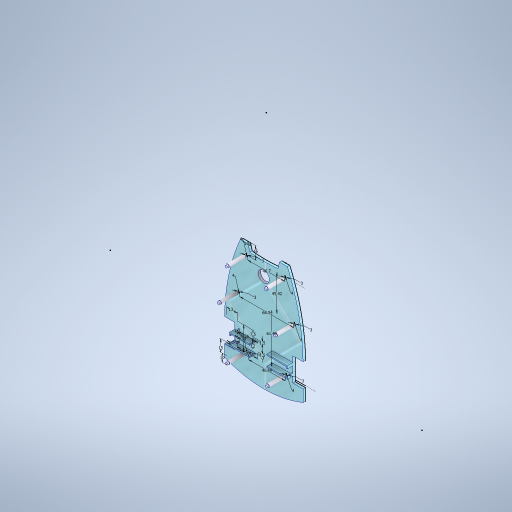
# Autodesk Inventor part: Part1
Saved by Autodesk Inventor 2024 (Build 280153000, 153)
## iProperties
Created: 2024-04-12
Part Number: Part1
Material: Generic
Document SubType Name: Modeling
Designer: Hitesh
Density: 1 g/cm^3
Appearance: Cool White
Author: Hitesh
Autodesk Inventor part; units mm, degrees
ref_plane "YZ Plane" through (0, 0, 0) normal (1, 0, 0) x (0, 1, 0)
ref_plane "XZ Plane" through (0, 0, 0) normal (0, 1, 0) x (-1, 0, 0)
ref_plane "XY Plane" through (0, 0, 0) normal (0, 0, 1) x (1, 0, 0)
sketch "Sketch1" plane through (0, 0, 0) normal (0, 0, 1) x (1, 0, 0)
  arc A0 (0, 10) -> (100, 10) centre (50, 130) ccw
  line L0 (0, 55) -> (13, 55)
  line L1 (13, 55) -> (13, 25)
  line L2 (13, 25) -> (0, 25)
  line L3 (13, 47.5) -> (39, 47.5)
  line L4 (39, 47.5) -> (39, 46)
  line L5 (39, 46) -> (13, 46)
  line L6 (13, 46) -> (13, 47.5)
  line L7 (13, 34) -> (39, 34)
  line L8 (39, 34) -> (39, 32.5)
  line L9 (39, 32.5) -> (13, 32.5)
  line L10 (13, 46) -> (14, 46)
  line L11 (14, 46) -> (14, 44)
  line L12 (14, 44) -> (13, 44)
  line L13 (13, 44) -> (13, 46)
  line L14 (13, 34) -> (14, 34)
  line L15 (14, 34) -> (14, 36)
  line L16 (14, 36) -> (13, 36)
  line L17 (13, 36) -> (13, 34)
  line L18 (30, 150) -> (32, 142)
  arc A1 (32, 142) -> (50, 141) centre (50, 303.5) ccw
  line L19 (100, 55) -> (87, 55)
  line L20 (87, 55) -> (87, 25)
  line L21 (87, 25) -> (100, 25)
  line L22 (87, 47.5) -> (61, 47.5)
  line L23 (61, 47.5) -> (61, 46)
  line L24 (61, 46) -> (87, 46)
  line L25 (87, 46) -> (87, 47.5)
  line L26 (61, 34) -> (61, 32.5)
  line L27 (87, 34) -> (61, 34)
  line L28 (61, 32.5) -> (87, 32.5)
  line L29 (87, 46) -> (86, 46)
  line L30 (86, 46) -> (86, 44)
  line L31 (86, 44) -> (87, 44)
  line L32 (87, 44) -> (87, 46)
  line L33 (87, 34) -> (86, 34)
  line L34 (86, 34) -> (86, 36)
  line L35 (86, 36) -> (87, 36)
  line L36 (87, 36) -> (87, 34)
  line L37 (70, 150) -> (68, 142)
  arc A2 (50, 141) -> (68, 142) centre (50, 303.5) ccw
  arc A3 (100, 55) -> (80, 150) centre (-148.869, 52.2118) ccw
  line L38 (70, 150) -> (80, 150)
  line L39 (20, 150) -> (30, 150)
  line L40 (100, 25) -> (100, 10)
  line L41 (0, 10) -> (0, 25)
  circle A4 centre (25.0045, 134) radius 1.5 construction
  circle A5 centre (74.7045, 134) radius 1.5 construction
  line L42 (16.9872, 134) -> (99.6032, 134) construction
  line L43 (12.0158, 134) -> (23.5045, 134)
  line L44 (74.7045, 134) -> (86.1932, 134)
  circle A6 centre (25.0045, 134) radius 2
  circle A7 centre (74.7045, 134) radius 2
  circle A8 centre (14.98, 88.58) radius 1.5 construction
  circle A9 centre (86.52, 88.58) radius 1.5 construction
  line L45 (16.652, 88.58) -> (99.2681, 88.58) construction
  line L46 (2.6559, 88.58) -> (13.48, 88.58)
  line L47 (86.52, 88.58) -> (97.3441, 88.58)
  circle A10 centre (14.98, 88.58) radius 2
  circle A11 centre (86.52, 88.58) radius 2
  line L48 (13, 50.0336) -> (87, 50.0336) construction
  line L49 (50, 50.0336) -> (50, 74.1687) construction
  arc A12 (20, 150) -> (0, 55) centre (248.869, 52.2118) ccw
  line L50 (0, 27.09) -> (23.905, 27.09)
  circle A13 centre (25.405, 27.09) radius 1.5 construction
  circle A14 centre (25.405, 27.09) radius 2
  circle A15 centre (76.095, 27.09) radius 1.5 construction
  circle A16 centre (76.095, 27.09) radius 2
  line L51 (30.9298, 27.09) -> (113.5459, 27.09) construction
  line L52 (76.095, 27.09) -> (100, 27.09)
  point P0 (0, 0)
  point P1 (75, 150)
  point P2 (50.8983, 94.4188)
  point P3 (62.5692, 16.9025)
  dimension "d68" = 3
  dimension "d74" = 3
  dimension "d80" = 3
  dimension "d10" = 10
  dimension "d12" = 30
  dimension "d13" = 13
  dimension "d14" = 15
  dimension "d15" = 26
  dimension "d16" = 1.5
  dimension "d19" = 26
  dimension "d20" = 1.5
  dimension "d23" = 7.5
  dimension "d24" = 12
  dimension "d25" = 1
  dimension "d26" = 2
  dimension "d27" = 1
  dimension "d28" = 2
  dimension "d35" = 10
  dimension "d69" = 3
  dimension "d70" = 46.7
  dimension "d71" = 16
  dimension "d72" = 4
  dimension "d73" = 4
  dimension "d75" = 3
  dimension "d76" = 68.54
  dimension "d77" = 4
  dimension "d78" = 4
  dimension "d79" = 45.42
  dimension "d81" = 3
  dimension "d83" = 4
  dimension "d84" = 4
  dimension "d86" = 61.49
  dimension "d107" = 46.69
  constraints: 106 end point, 23 horizontal, 23 point on line, 14 centre point, 13 point on circle, 11 vertical, 8 parallel, 7 perpendicular, 6 coincident, 4 collinear, 3 horizontal alignment, 1 midpoint, 1 symmetric about line, 31 other
  measures "d10" distance of L41.start point (0, 0)
  measures "d12" distance of L0.end L1.end
  measures "d13" distance of L0.start L0.end
  measures "d14" distance from line of L41.start L2
  measures "d15" distance of L4.end L5.end
  measures "d16" distance of L3.end L4.end
  measures "d19" distance of L8.end L9.end
  measures "d20" distance of L8.start L8.end
  measures "d23" distance between parallel lines of L0 L3
  measures "d24" distance between parallel lines of L7 L5
  measures "d25" distance of L11.end L12.end
  measures "d26" distance of L10.end L11.end
  measures "d27" distance of L16.end L15.end
  measures "d28" distance of L15.end L14.end
  measures "d35" distance of L39.start L18.start
  measures "d69" diameter of A5
  measures "d71" distance from line of point (25.005, 134) L39
  measures "d72" diameter of A6
  measures "d73" diameter of A7
  measures "d75" diameter of A9
  measures "d77" diameter of A10
  measures "d78" diameter of A11
  measures "d79" distance between parallel lines of L45 L42
  measures "d81" diameter of A15
  measures "d83" diameter of A14
  measures "d84" diameter of A16
  measures "d86" distance between parallel lines of L51 L45
extrude "Extrusion1" add sketch "Sketch1" along normal blind 10 contours L1 L7 L8 L9 | L28 L26 L27 L20 | L1 L16 L15 L7 | L27 L34 L35 L20 | L1 L5 L11 L12 | L31 L30 L24 L20 | L1 L3 L4 L5 | L24 L23 L22 L20
extrude "Extrusion3" add sketch "Sketch1" along normal blind 3 contours L41 L2 L1 L9 L8 L7 L15 L16 L12 L11 L5 L4 L3 L0 A12 L39 L18 A1 A2 L37 L38 A3 L19 L20 L22 L23 L24 L30 L31 L35 L34 L27 L26 L28 L21 L40 A0
sketch "Sketch2" plane through (0, 0, 3) normal (0, 0, 1) x (1, 0, 0)
  line L0 (39, 34) -> (14, 34) projected
  line L1 (17.3, 34) -> (16.3, 34)
  line L2 (16.3, 34) -> (16.3, 36)
  line L3 (16.3, 36) -> (17.3, 36)
  line L4 (17.3, 36) -> (17.3, 34)
  line L5 (14, 34) -> (14, 36) projected
  line L6 (61, 46) -> (86, 46) projected
  line L7 (83.7, 46) -> (82.7, 46)
  line L8 (82.7, 46) -> (82.7, 44)
  line L9 (82.7, 44) -> (83.7, 44)
  line L10 (83.7, 44) -> (83.7, 46)
  line L11 (86, 46) -> (86, 44) projected
  point P0 (0, 0)
  point P1 (14, 35)
  dimension "d89" = 1
  dimension "d90" = 2
  dimension "d91" = 2.3
  dimension "d92" = 1
  dimension "d93" = 2
  dimension "d94" = 2.3
  constraints: 16 end point, 4 parallel, 2 horizontal, 2 perpendicular, 2 point on line, 1 midpoint
  measures "d89" distance of L2.end L3.end
  measures "d90" distance of L1.end L2.end
  measures "d91" distance from line of point (14, 35) L2
  measures "d92" distance of L9.end L8.end
  measures "d93" distance of L8.end L7.end
  measures "d94" distance between parallel lines of L10 L11
extrude "Extrusion4" add sketch "Sketch2" along normal blind 1.5
extrude "Extrusion5" add sketch "Sketch1" along normal blind 24 contours A16 | A11 | A7 | A6 | A10 | A14
sketch "Sketch4" plane through (74.7045, 134, 24) normal (0, 0, 1) x (1, 0, 0)
  circle A0 centre (-49.7, 0) radius 2 projected
  circle A1 centre (-49.7, 0) radius 1.5
  circle A2 centre (0, 0) radius 2 projected
  circle A3 centre (0, 0) radius 1.5
  circle A4 centre (-59.7245, -45.42) radius 2 projected
  circle A5 centre (-59.7245, -45.42) radius 1.5
  circle A6 centre (11.8155, -45.42) radius 2 projected
  circle A7 centre (11.8155, -45.42) radius 1.5
  circle A8 centre (1.3905, -106.91) radius 2 projected
  circle A9 centre (1.3905, -106.91) radius 1.5
  circle A10 centre (-49.2995, -106.91) radius 2 projected
  circle A11 centre (-49.2995, -106.91) radius 1.5
  point P0 (-74.7045, -134)
  dimension "d99" = 3
  dimension "d100" = 3
  dimension "d101" = 3
  dimension "d102" = 3
  dimension "d103" = 3
  dimension "d104" = 3
  constraints: 6 centre point, 6 coincident
  measures "d99" diameter of A1
  measures "d100" diameter of A3
  measures "d101" diameter of A5
  measures "d102" diameter of A7
  measures "d103" diameter of A9
  measures "d104" diameter of A11
extrude "Extrusion6" add sketch "Sketch4" along normal blind 2 contours A1 | A3 | A5 | A7 | A9 | A11
sketch "Sketch5" plane through (0, 0, 3) normal (0, 0, 1) x (1, 0, 0)
  circle A0 centre (50, 124.26) radius 7
  point P0 (0, 0)
  dimension "d108" = 14
  constraints: 1 centre point
  measures "d108" diameter of A0
extrude "Extrusion7" cut sketch "Sketch5" against normal blind 10
body "Solid1"
